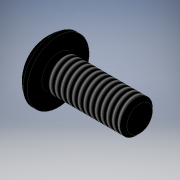
# Autodesk Inventor part: 11-4310
Saved by Autodesk Inventor 2025 (Build 290162000, 162)
## iProperties
Created: 2024-04-27
Part Number: 11-4310
Material: Generic
Catalog Web Link: www.cadenas.de
Description: 11-4310, 11-4312-Button Head Socket Cap Screws
Vendor: 8020
Document SubType Name: Modeling
Designer: psAdmin
Manufacturer: 8020
Mass: 0.184692 g
Surface Area: 2.54318 cm^2
Volume: 0.184692 cm^3
Density: 1 g/cm^3
Appearance: PSOLRGB-0-0-0
Category: PARTsolutions
Company: 8020
PSOL_IDENT_0: {$CADENAS_DATA/23d-libs/8020/metric/fastening_options/11_4310.prj},166 {VTYP=3D},{NB=11-4310},{LINA=
PSOL_IDENT_1: 11-4310},{NN=11-4310, 11-4312},{DATE=27.07.2023 20:18:57},{GEOMDATE=28.08.2012 10:43:00},{VERSION=},
PSOL_IDENT_2: {LINEID=40},{WBVAR=L},{WBNUMERIC=L}  {NB=11-4310},{LINA=11-4310},{KT=DUMMY},{PN=11-4310},{THRD=M4 x
PSOL_IDENT_3: 0.7},{FIN=Black-Coated},{M=4},{L=10},{L1=10,12},{A=7.6},{B=2.5},{C=1.87},{E=2.19}
NB: 11-4310
NN: 11-4310, 11-4312
NT: Button Head Socket Cap Screws
NBSYN: $PN.
LINA: 11-4310
CATALOG: 80/20
PN: 11-4310
THRD: M4 x 0.7
FIN: Black-Coated
L: 10
A: 7.6
B: 2.5
E: 2.19
SUPPLIER: 8020
ARTICLENO: 11-4310
BOMINFO: 11-4310
CREATOR: CADENAS GmbH
Title: 11-4310
Author: Cadenas PARTsolutions
Comments: Button Head Socket Cap Screws
Autodesk Inventor part; units mm, degrees
sketch "Sketch_1" plane through (0, 0, 0) normal (0, 0, 1) x (1, 0, 0)
  line L0 (10, 0) -> (0.4017, 0)
  line L1 (0.4017, 0) -> (-0.32, 1.25)
  line L2 (-0.32, 1.25) -> (-2.19, 1.25)
  line L3 (-2.19, 1.25) -> (-2.19, 1.5)
  arc A0 (-0.5, 3.8) -> (-2.19, 1.5) centre (1.4931, 0.5646) ccw
  line L4 (-0.5, 3.8) -> (0, 3.8)
  line L5 (0, 3.8) -> (0, 2)
  line L6 (0, 2) -> (9.5705, 2)
  line L7 (9.5705, 2) -> (10, 1.5705)
  line L8 (10, 1.5705) -> (10, 0)
  line L9 (10, 0) -> (0.4017, 0)
  constraints: 20 end point, 2 point on circle, 1 centre point
revolve "Revolution1" add sketch "Sketch_1" angle 360 about axis through (10, 0, 0) along (1, 0, 0)
thread "Thread1" size "M4x0.7" class "6g" standard "ISO Metric profile" length 8.8266
sketch "Sketch_2" plane through (-2.19, 0, 0) normal (1, 0, 0) x (0, 0, -1)
  line L0 (-1.25, -0.7217) -> (0, -1.4434)
  line L1 (0, -1.4434) -> (1.25, -0.7217)
  line L2 (1.25, -0.7217) -> (1.25, 0.7217)
  line L3 (1.25, 0.7217) -> (0, 1.4434)
  line L4 (0, 1.4434) -> (-1.25, 0.7217)
  line L5 (-1.25, 0.7217) -> (-1.25, -0.7217)
  constraints: 12 end point
extrude "Extrusion1" cut sketch "Sketch_2" along normal blind 1.87
ref_plane "screw_XY" through (0, 0, 0) normal (1, 0, 0) x (0, 0, -1)
ref_plane "screw_YZ" through (0, 0, 0) normal (0, 0, -1) x (0, 1, 0)
ref_plane "screw_ZX" through (0, 0, 0) normal (0, 1, 0) x (1, 0, 0)
body "Solid1"
